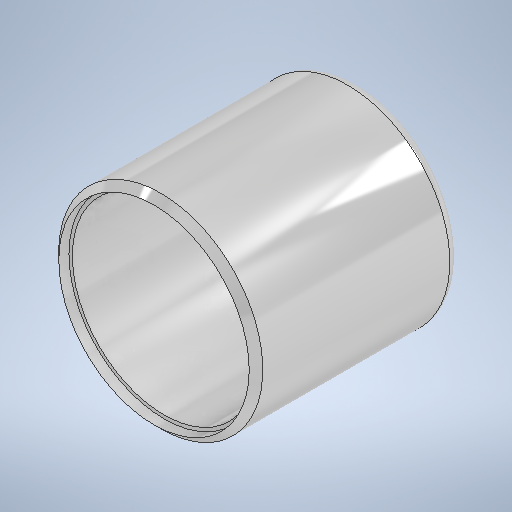
# Autodesk Inventor part: Plenum
Saved by Autodesk Inventor 2025.2 (Build 292293000, 293)
## iProperties
Created: 2026-06-25
Part Number: Plenum
Material: Generic
Document SubType Name: Modeling
Designer: Simon
Density: 1 g/cm^3
Appearance: Aluminum - Polished
Author: Simon
Autodesk Inventor part; units mm, degrees
ref_plane "YZ Plane" through (0, 0, 0) normal (1, 0, 0) x (0, 1, 0)
ref_plane "XZ Plane" through (0, 0, 0) normal (0, 1, 0) x (-1, 0, 0)
ref_plane "XY Plane" through (0, 0, 0) normal (0, 0, 1) x (1, 0, 0)
sketch "Sketch2" plane through (0, 0, 0) normal (1, 0, 0) x (0, 1, 0)
  line L0 (0, 0) -> (30, 0)
  line L1 (30, 60) -> (30, -60)
  line L2 (30, 60) -> (27, 60)
  line L3 (27, 60) -> (27, -60)
  line L4 (27, -60) -> (30, -60)
  line L5 (27, 60) -> (0, 60)
  line L6 (0, 60) -> (0, 60)
  line L7 (0, 60) -> (0, 54)
  line L8 (0, 54) -> (27, 54)
  line L9 (27, -60) -> (0, -60)
  line L10 (0, -60) -> (0, -60)
  line L11 (0, -60) -> (0, -54)
  line L12 (0, -54) -> (27, -54)
  line L13 (0, 60) -> (0, -60)
  line L14 (27, 0) -> (28, 0)
  line L15 (28, 0) -> (28, -3)
  line L16 (28, -3) -> (27, -3)
  line L17 (28, 0) -> (28, 2)
  line L18 (28, 2) -> (30, 2)
  line L19 (30, 2) -> (28, 0)
  line L20 (28, 0) -> (28, -2)
  line L21 (28, -2) -> (30, -2)
  line L22 (30, -2) -> (28, 0)
  dimension "d12" = 30
  dimension "d13" = 120
  dimension "d14" = 3
  dimension "d15" = 0
  dimension "d16" = 6
  dimension "d17" = 6
  dimension "d26" = 1
  dimension "d27" = 3
  dimension "d28" = 2
  dimension "d29" = 2
  constraints: 46 end point, 13 point on line, 8 perpendicular, 2 horizontal, 2 midpoint, 2 parallel, 2 vertical
  measures "d12" distance of L0.start L0.end
  measures "d13" distance of L1.start L1.end
  measures "d14" distance of L1.start L2.end
  measures "d15" distance of L5.end L6.end
  measures "d16" distance of L6.end L7.end
  measures "d17" distance of L10.end L11.end
  measures "d26" distance of L14.start L14.end
  measures "d27" distance of L14.end L15.end
  measures "d28" distance of L14.end L17.end
  measures "d29" distance of L14.end L20.end
revolve "Revolution1" add sketch "Sketch2" angle 360 about axis through (0, 0, 60) along (0, 0, -1) contours L12 L3 L9 L11 | L22 L21 L15 | L16 L15 L21 L1 L4 L3
fillet "Fillet2" radius 3 1 edges at (0, -30, -60)
fillet "Fillet3" radius 3 1 edges at (0, -27, -54)
sketch "Sketch3" plane through (0, 0, -60) normal (0, 0, -1) x (-1, 0, 0)
  point P0 (0, 0)
  point P1 (0, 0)
  constraints: 1 coincident
hole "Hole1" at (0, 0, -60) direction (0, 0, 1) diameter 7.9502 end through all taper from width 8.7366 to width 8.304 over 6.924 thread size "1/8" designation "1/8 - 27 NPT" standard "NPT"
chamfer "Chamfer3" distance 0.5 angle 45 1 edges at (0, -4.3683, -60)
body "Solid2"
